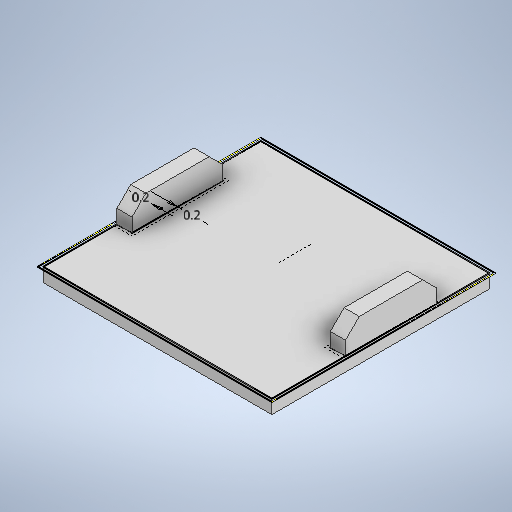
# Autodesk Inventor part: tapita
Saved by Autodesk Inventor 2025.1 (Build 291241020, 241B)
## iProperties
Created: 2024-12-17
Part Number: tapita
Material: Genérico
Document SubType Name: Modeling
Designer: ctamashiro
Density: 1 g/cm^3
Appearance: Valor por defecto
Author: ctamashiro
Autodesk Inventor part; units mm, degrees
ref_plane "YZ Plane" through (0, 0, 0) normal (1, 0, 0) x (0, 1, 0)
ref_plane "XZ Plane" through (0, 0, 0) normal (0, 1, 0) x (-1, 0, 0)
ref_plane "XY Plane" through (0, 0, 0) normal (0, 0, 1) x (1, 0, 0)
sketch "Boceto1" plane through (0, 0, 0) normal (0, 1, 0) x (-1, 0, 0)
  line L0 (-7, 3.5) -> (-8.5, 3.5)
  line L1 (-7, -3.5) -> (-7, 3.5)
  line L2 (-8.5, -3.5) -> (-7, -3.5)
  line L3 (-8.5, -3.5) -> (-8.5, -7.3536)
  line L4 (-8.5, -7.3536) -> (8.5, -7.3536)
  line L5 (8.5, -7.3536) -> (8.5, -3.5)
  line L6 (7, -3.5) -> (8.5, -3.5)
  line L7 (7, 3.5) -> (7, -3.5)
  line L8 (8.5, 3.5) -> (7, 3.5)
  line L9 (8.5, 3.5) -> (8.5, 8.8489)
  line L10 (-8.5, 8.8489) -> (8.5, 8.8489)
  line L11 (-8.5, 8.8489) -> (-8.5, 3.5)
  circle A0 centre (0, 0) radius 5.5
  point P0 (-1.5892, 6.097)
  point P1 (-7, 0)
  dimension "d26" = 16.2026
  dimension "d27" = 17
  dimension "d28" = 5.3489
  dimension "d29" = 7
  dimension "d30" = 11
  dimension "d31" = 8.8489
  dimension "d32" = 8.5
  dimension "d34" = 1.5
  dimension "d35" = 1.5
  constraints: 24 end point, 6 parallel, 4 collinear, 1 centre point, 1 coincident, 1 horizontal, 1 midpoint, 1 perpendicular, 1 vertical
  measures "d26" distance between parallel lines of L4 L10
  measures "d27" distance of L10.start L9.end
  measures "d28" distance of L10.start L0.end
  measures "d29" distance between parallel lines of L2 L0
  measures "d30" diameter of A0
  measures "d31" distance from line of L10 A0.centre
  measures "d32" distance from line of L3 A0.centre
  measures "d34" distance between parallel lines of L11 L1
  measures "d35" distance between parallel lines of L7 L9
sketch "Boceto2" plane through (0, 0, 0) normal (0, 1, 0) x (-1, 0, 0)
  line L0 (8.5, 3.5) -> (7, 3.5) construction
  line L1 (7, 3.5) -> (7, -3.5) construction
  line L2 (7, -3.5) -> (8.5, -3.5) construction
  line L3 (-7, 3.5) -> (-8.5, 3.5) construction
  line L4 (-7, -3.5) -> (-7, 3.5) construction
  line L5 (-8.5, -3.5) -> (-7, -3.5) construction
  line L6 (-8.5, -3.5) -> (-8.5, -7.3536) construction
  line L7 (-8.5, 8.8489) -> (-8.5, 3.5) construction
  line L8 (8.5, 3.5) -> (8.5, 8.8489) construction
  line L9 (8.5, -7.3536) -> (8.5, -3.5) construction
  line L10 (7, 3.5) -> (8.5, 3.5) construction
  line L11 (8.5, 3.5) -> (8.5, -3.5) construction
  line L12 (8.5, -3.5) -> (7, -3.5) construction
  line L13 (7, -3.5) -> (7, 3.5) construction
  line L14 (-8.5, 3.5) -> (-7, 3.5) construction
  line L15 (-7, 3.5) -> (-7, -3.5) construction
  line L16 (-7, -3.5) -> (-8.5, -3.5) construction
  line L17 (-8.5, -3.5) -> (-8.5, 3.5) construction
  line L18 (7.2, 3.3) -> (8.3, 3.3)
  line L19 (8.3, 3.3) -> (8.3, -3.3)
  line L20 (8.3, -3.3) -> (7.2, -3.3)
  line L21 (7.2, -3.3) -> (7.2, 3.3)
  line L22 (8.5, 8.8489) -> (-8.5, 8.8489)
  line L23 (-8.5, 8.8489) -> (-8.5, -7.3536)
  line L24 (-8.5, -7.3536) -> (8.5, -7.3536)
  line L25 (8.5, -7.3536) -> (8.5, 8.8489)
  line L26 (0, 0) -> (0, -2.5786) construction
  line L27 (-7.2, 3.3) -> (-8.3, 3.3)
  line L28 (-8.3, 3.3) -> (-8.3, -3.3)
  line L29 (-8.3, -3.3) -> (-7.2, -3.3)
  line L30 (-7.2, -3.3) -> (-7.2, 3.3)
  line L31 (8.3, 8.6489) -> (-8.3, 8.6489)
  line L32 (-8.3, 8.6489) -> (-8.3, -7.1536)
  line L33 (-8.3, -7.1536) -> (8.3, -7.1536)
  line L34 (8.3, -7.1536) -> (8.3, 8.6489)
  dimension "d36" = 0.2
  dimension "d41" = 0.2
  constraints: 50 end point, 10 parallel, 5 perpendicular, 4 symmetric about line, 3 horizontal, 1 vertical, 6 other
  measures "d36" distance between parallel lines of L13 L21
  measures "d41" distance between parallel lines of L25 L34
extrude "Extrusión1" add sketch "Boceto2" against normal blind 1 contours L21 L20 L34 L33 L32 L29 L30 L27 L31 L18 | L18 L19 L20 L21 | L27 L30 L29 L28
extrude "Extrusión2" add sketch "Boceto2" along normal blind 2 contours L18 L19 L20 L21 | L27 L30 L29 L28
chamfer "Chaflán1" distance 1 angle 45 4 edges at (-7.75, 2, 3.3) (-7.75, 2, -3.3) (7.75, 2, 3.3) (7.75, 2, -3.3)
equation "\"d35\" = d34"
